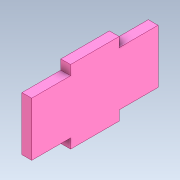
# Autodesk Inventor part: FrontWall
Saved by Autodesk Inventor 2021 (Build 250183000, 183)
## iProperties
Created: 2021-08-31
Part Number: FrontWall
Material: ABS Plastic
Document SubType Name: Modeling
Designer: digge
Density: 1.06 g/cm^3
Appearance: Pink
Author: digge
Autodesk Inventor part; units mm, degrees
ref_plane "YZ Plane" through (0, 0, 0) normal (1, 0, 0) x (0, 1, 0)
ref_plane "XZ Plane" through (0, 0, 0) normal (0, 1, 0) x (-1, 0, 0)
ref_plane "XY Plane" through (0, 0, 0) normal (0, 0, 1) x (1, 0, 0)
sketch "Sketch1" plane through (0, 0, 0) normal (1, 0, 0) x (0, 1, 0)
  line L0 (105.4, 211.9879) -> (50, 211.9879)
  line L1 (50, 211.9879) -> (50, 171.9879)
  line L2 (50, 171.9879) -> (40, 171.9879)
  line L3 (40, 171.9879) -> (40, 121.9879)
  line L4 (40, 121.9879) -> (50, 121.9879)
  line L5 (50, 121.9879) -> (50, 81.9879)
  line L6 (50, 81.9879) -> (105.4, 81.9879)
  line L7 (105.4, 81.9879) -> (105.4, 121.9879)
  line L8 (105.4, 121.9879) -> (115.4, 121.9879)
  line L9 (115.4, 121.9879) -> (115.4, 171.9879)
  line L10 (115.4, 171.9879) -> (105.4, 171.9879)
  line L11 (105.4, 211.9879) -> (105.4, 171.9879)
  line L12 (40, 146.9879) -> (115.4, 146.9879) construction
  point P0 (0, 0)
  dimension "d0" = 10
  dimension "d1" = 10
  dimension "d2" = 50
  dimension "d3" = 55.4
  dimension "d4" = 130
  constraints: 26 end point, 8 perpendicular, 6 point on line, 2 midpoint, 1 horizontal, 1 other
  measures "d0" distance of L1.end L2.end
  measures "d1" distance of L9.end L10.end
  measures "d2" distance of L8.end L9.end
  measures "d3" distance of L0.start L0.end
  measures "d4" distance between parallel lines of L6 L0
extrude "Extrusion1" add sketch "Sketch1" along normal blind 10
equation "\"d0\" = Width"
equation "\"d1\" = Width"
equation "\"d5\" = Width"
equation "\"Width\" = 10"
body "Solid1"
